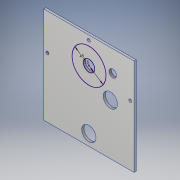
# Autodesk Inventor part: 板2
Saved by Autodesk Inventor 2019 (Build 230136000, 136)
## iProperties
Created: 2020-09-28
Part Number: 板2
Material: アルミニウム 6061
Document SubType Name: Modeling
Designer: zhept
Density: 2.7 g/cm^3
Appearance: アルミニウム - フラット
Mass: 128.079 g
Surface Area: 338.754 cm^2
Volume: 47.4367 cm^3
Author: zhept
Autodesk Inventor part; units mm, degrees
ref_plane "YZ Plane" through (0, 0, 0) normal (1, 0, 0) x (0, 1, 0)
ref_plane "XZ Plane" through (0, 0, 0) normal (0, 1, 0) x (-1, 0, 0)
ref_plane "XY Plane" through (0, 0, 0) normal (0, 0, 1) x (1, 0, 0)
sketch "スケッチ3" plane through (0, 0, 0) normal (0, 0, 1) x (1, 0, 0)
  line L0 (60, -99.3436) -> (-60, -99.3436)
  line L1 (-60, -99.3436) -> (-60, 99.3436)
  line L2 (-60, 99.3436) -> (60, 99.3436)
  line L3 (60, 99.3436) -> (60, -99.3436)
  line L4 (60, -99.3436) -> (-60, 99.3436) construction
  line L5 (-60, -99.3436) -> (60, 99.3436) construction
  point P0 (0, 0)
  dimension "d25" = 120
  constraints: 12 end point, 2 midpoint, 2 parallel, 1 horizontal, 1 perpendicular
  measures "d25" distance of L0.start L0.end
extrude "押し出し1" add sketch "スケッチ3" against normal blind 3
sketch "スケッチ4" plane through (0, 0, 0) normal (0, 0, 1) x (1, 0, 0)
  line L0 (0, 45.0711) -> (68.3595, 45.0711)
  line L1 (68.3595, 45.0711) -> (-74.3824, 45.0711)
  line L2 (-74.3824, 45.0711) -> (108.1656, 45.0711)
  line L3 (108.1656, 45.0711) -> (108.1656, 129.4154)
  line L4 (108.1656, 129.4154) -> (-74.3824, 129.4154)
  line L5 (-74.3824, 129.4154) -> (-74.3824, 45.0711)
  point P0 (0, 0)
  constraints: 12 end point, 2 horizontal, 2 parallel, 1 perpendicular, 1 point on line
extrude "押し出し4" cut sketch "スケッチ4" against normal blind 10
sketch "スケッチ12" plane through (0, 0, 0) normal (0, 0, 1) x (1, 0, 0)
  circle A0 centre (0, 0) radius 7.5
  circle A1 centre (0, 0) radius 22.5
  dimension "d85" = 15
  dimension "d93" = 45
  constraints: 2 centre point, 2 coincident
  measures "d85" diameter of A0
  measures "d93" diameter of A1
sketch "スケッチ13" plane through (0, 0, 0) normal (0, 0, 1) x (1, 0, 0)
  circle A0 centre (0, 0) radius 7.5
  circle A1 centre (0, 0) radius 32.5
  circle A2 centre (31.7707, 6.8465) radius 25
  circle A3 centre (31.7707, 6.8465) radius 7.5
  circle A4 centre (31.7707, 6.8465) radius 32.5
  circle A5 centre (28.5436, -25.4929) radius 25
  circle A6 centre (28.5436, -25.4929) radius 20
  circle A7 centre (28.5436, -25.4929) radius 60
  circle A8 centre (0, -78.2685) radius 40
  circle A9 centre (0, -78.2685) radius 50
  circle A10 centre (31.7707, 6.8465) radius 5
  circle A11 centre (28.5436, -25.4929) radius 9.5
  circle A12 centre (0, -78.2685) radius 9.5
  dimension "d87" = 65
  dimension "d89" = 65
  dimension "d91" = 120
  dimension "d86" = 15
  dimension "d88" = 15
  dimension "d90" = 40
  dimension "d92" = 100
  dimension "d96" = 10
  dimension "d97" = 19
  dimension "d98" = 19
  constraints: 10 centre point, 10 coincident, 3 tangent, 9 other
  measures "d86" diameter of A0
  measures "d88" diameter of A3
  measures "d90" diameter of A6
  measures "d92" diameter of A9
  measures "d96" diameter of A10
  measures "d97" diameter of A11
  measures "d98" diameter of A12
extrude "押し出し15" cut sketch "スケッチ12" against normal blind 10 contours A0
extrude "押し出し16" cut sketch "スケッチ13" against normal blind 10 contours A10 A1 | A1 A10 | A11 A1 A2 | A2 A1 A4 A11 | A4 A1 A11 | A2 A11 A4 A1 | A1 A11 A2 | A4 A11 A1 | A12 A7 | A7 A12
sketch "スケッチ14" plane through (0, 0, 0) normal (0, 0, 1) x (1, 0, 0)
  line L0 (-60, -99.3436) -> (-60, 45.0711) projected
  line L1 (60, 45.0711) -> (60, -99.3436) projected
  line L2 (-60, 45.0711) -> (60, 45.0711)
  line L3 (60, 45.0711) -> (60, -92.9289)
  line L4 (60, -92.9289) -> (-60, -92.9289)
  line L5 (-60, -92.9289) -> (-60, 45.0711)
  point P0 (0, 0)
  dimension "d101" = 138
  constraints: 8 end point, 2 parallel, 1 horizontal, 1 perpendicular, 1 point on line
  measures "d101" distance of L2.end L3.end
extrude "押し出し17" cut sketch "スケッチ14" against normal blind 10 keep common part
sketch "スケッチ15" plane through (-60, 45.0711, 0) normal (0, 1, 0) x (1, 0, 0)
  line L0 (-15.5399, 21.7204) -> (138.9638, 21.7204)
  line L1 (138.9638, 21.7204) -> (138.9638, -41.1938)
  line L2 (138.9638, -41.1938) -> (-15.5399, -41.1938)
  line L3 (-15.5399, -41.1938) -> (-15.5399, 21.7204)
  point P0 (60, 0)
  constraints: 8 end point, 2 parallel, 1 horizontal, 1 perpendicular
extrude "押し出し18" cut sketch "スケッチ15" against normal blind 10
sketch "スケッチ16" plane through (0, 0, 0) normal (0, 0, 1) x (1, 0, 0)
  circle A0 centre (31.7707, 6.8465) radius 5 projected
  circle A1 centre (31.7707, 6.8465) radius 25
  circle A2 centre (28.5436, -25.4929) radius 9.5 projected
  circle A3 centre (28.5436, -25.4929) radius 25
  circle A4 centre (55, -13) radius 2
  circle A5 centre (-55, -13) radius 2
  circle A6 centre (0, 29) radius 2
  point P0 (0, 0)
  dimension "d109" = 50
  dimension "d110" = 50
  dimension "d111" = 4
  dimension "d112" = 4
  dimension "d113" = 4
  constraints: 5 centre point, 2 coincident
  measures "d109" diameter of A1
  measures "d110" diameter of A3
  measures "d111" diameter of A4
  measures "d112" diameter of A5
  measures "d113" diameter of A6
extrude "押し出し19" cut sketch "スケッチ16" against normal blind 10 contours A4 | A5 | A6
